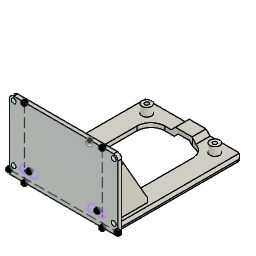
CPU Mount - Blank (Autodesk Fusion 360 design; units mm, degrees)
Autodesk Fusion 360 part; units mm, degrees
note: some values were not read from the file. Set by a fixed rule: which sketch regions a step uses.
sketch "Sketch3" plane through (0, 0, 0) normal (0, 1, 0) x (1, 0, 0)
  line L0 (-39, -50) -> (39, -50)
  line L1 (39, -50) -> (39, 0)
  line L2 (39, 0) -> (-39, 0)
  line L3 (-39, 0) -> (-39, -50)
  line L4 (-56.129, 0) -> (56.129, 0) construction
  circle A0 centre (-36, -47) radius 1.7
  circle A1 centre (-36, -47) radius 3
  circle A2 centre (36, -47) radius 1.7
  circle A3 centre (36, -47) radius 3
  circle A4 centre (-36, -6.7) radius 1.7
  circle A5 centre (-36, -6.7) radius 3
  circle A6 centre (36, -6.7) radius 1.7
  circle A7 centre (36, -6.7) radius 3
  line L5 (-39, -5) -> (39, -5) construction
  dimension "d32" = 50
  dimension "d33" = 78
  dimension "d34" = 39
  dimension "d35" = 3.4
  dimension "d36" = 6
  dimension "d37" = 3.4
  dimension "d38" = 6
  dimension "d39" = 3.4
  dimension "d40" = 6
  dimension "d41" = 3.4
  dimension "d42" = 6
  dimension "d43" = 5
  constraint horizontal L0
  constraint vertical L1
  constraint horizontal L2
  constraint vertical L3
  constraint perpendicular L3 L4
  constraint midpoint origin L4
  constraint collinear L2 L4
  constraint concentric A0 A1
  constraint concentric A2 A3
  constraint concentric A4 A5
  constraint concentric A6 A7
  constraint horizontal A0.centre A2.centre
  constraint vertical A2.centre A6.centre
  constraint vertical A0.centre A4.centre
  constraint horizontal A4.centre A6.centre
  constraint tangent L0 A1
  constraint tangent L3 A1
  constraint tangent L1 A3
  constraint coincident L3 L5.start
  constraint coincident L1 L5.end
  constraint perpendicular L1 L5
  constraint tangent A6 L5
  measures "d32" distance of L0.start L2.end
  measures "d33" distance of L0.start L0.end
  measures "d34" distance of origin L3
  measures "d35" diameter of A0
  measures "d36" diameter of A1
  measures "d37" diameter of A2
  measures "d38" diameter of A3
  measures "d39" diameter of A4
  measures "d40" diameter of A5
  measures "d41" diameter of A6
  measures "d42" diameter of A7
  measures "d43" distance of L1.end L5.end
extrude "Extrude3" add sketch "Sketch3" along normal blind 3 contours A7 | A5 | L0 L1 L2 L3 A1 A3 | A1 | A3
sketch "Sketch4" plane through (0, 3, 0) normal (0, 1, 0) x (-1, 0, 0)
  circle A0 centre (36, 47) radius 1.7
  circle A1 centre (36, 6.7) radius 1.7
  circle A2 centre (-36, 47) radius 1.7
  circle A3 centre (-36, 6.7) radius 1.7
  line L0 (36, 50) -> (-36, 50)
  arc A4 (-36, 50) -> (-39, 47) centre (-36, 47) ccw
  line L1 (-39, 47) -> (-39, 0)
  line L2 (-39, 0) -> (39, 0)
  line L3 (39, 0) -> (39, 47)
  arc A5 (39, 47) -> (36, 50) centre (36, 47) ccw
  line L4 (-39, 3) -> (39, 3) construction
  line L5 (-35.6, 3) -> (35.6, 3)
  line L6 (35.6, 3) -> (35.6, 0)
  line L7 (35.6, 0) -> (-35.6, 0)
  line L8 (-35.6, 0) -> (-35.6, 3)
  line L9 (0, 50) -> (0, 0) construction
  line L10 (35.6, 1.2) -> (33.8, 3)
  line L11 (35.6, 1.2) -> (38.7868, 1.2) construction
  line L12 (-35.6, 1.2) -> (-33.8, 3)
  line L13 (-35.6, 1.2) -> (-32.9375, 1.2) construction
  point P0 (0, 3)
  dimension "d46" = 3
  dimension "d47" = 71.2
  dimension "d48" = 135
  dimension "d49" = 1.2
  dimension "d50" = 45
  dimension "d51" = 1.2
  constraint coincident L1 L4.start
  constraint coincident L3 L4.end
  constraint perpendicular L3 L4
  constraint horizontal L5
  constraint vertical L6
  constraint horizontal L7
  constraint vertical L8
  constraint midpoint L0 L9.start
  constraint coincident L9.end origin
  constraint midpoint L5 P0
  constraint coincident L9 P0
  constraint collinear L2 L7
  constraint collinear L4 L5
  constraint horizontal L11
  constraint coincident L6 L10.start
  constraint coincident L5 L10.end
  constraint horizontal L13
  constraint coincident L8 L12.start
  constraint coincident L4 L12.end
  measures "d46" distance of L2.end L4.end
  measures "d47" distance of L5.start L5.end
  measures "d48" angle of L10 L11
  measures "d49" distance of L6.end L10.start
  measures "d50" angle of L12 L13
  measures "d51" distance of L7.end L12.start
extrude "Extrude4" add sketch "Sketch4" along normal blind 90 contours L2 L5 L6 L7 L8 L10 L12
sketch "Sketch5" plane through (0, 0, 3) normal (0, 0, 1) x (-1, 0, 0)
  line L0 (33.8, -3) -> (-33.8, -3)
  line L1 (-33.8, -3) -> (-33.8, -93)
  line L2 (-33.8, -93) -> (33.8, -93)
  line L3 (33.8, -93) -> (33.8, -3)
  line L4 (0, -3) -> (0, -93) construction
  circle A0 centre (24.5, -26.5) radius 1.45
  circle A1 centre (24.5, -26.5) radius 3.5
  circle A2 centre (24.5, -84.5) radius 1.45
  circle A3 centre (24.5, -84.5) radius 3.5
  circle A4 centre (-24.5, -26.5) radius 1.45
  circle A5 centre (-24.5, -26.5) radius 3.5
  circle A6 centre (-24.5, -84.5) radius 1.45
  circle A7 centre (-24.5, -84.5) radius 3.5
  line L5 (28, -3) -> (-28, -3)
  line L6 (-28, -3) -> (-28, -88) construction
  line L7 (-28, -88) -> (28, -88) construction
  line L8 (28, -88) -> (28, -3) construction
  line L9 (20, -13) -> (-20, -13)
  line L10 (-20, -13) -> (-20, -83)
  line L11 (-20, -83) -> (20, -83)
  line L12 (20, -83) -> (20, -13)
  line L13 (33.8, -48) -> (-33.8, -48) construction
  line L14 (-28.5, -3) -> (-31.5, -3)
  line L15 (-31.5, -3) -> (-31.5, -29)
  line L16 (-31.5, -29) -> (-28.5, -29)
  line L17 (-28.5, -29) -> (-28.5, -3)
  point P0 (0, -88)
  point P1 (-28, -3)
  point P2 (0, -13)
  point P3 (20, -48)
  point P4 (-33.8, -48)
  point P5 (33.8, -48)
  dimension "d54" = 2.9
  dimension "d55" = 7
  dimension "d56" = 2.9
  dimension "d57" = 7
  dimension "d58" = 2.9
  dimension "d59" = 7
  dimension "d60" = 2.9
  dimension "d61" = 7
  dimension "d62" = 58
  dimension "d63" = 49
  dimension "d64" = 23.5
  dimension "d70" = 56
  dimension "d71" = 85
  dimension "d86" = 70
  dimension "d87" = 70
  dimension "d88" = 40
  dimension "d159" = 3
  dimension "d160" = 26
  dimension "d161" = 7
  constraint midpoint L0 L4.start
  constraint midpoint L2 L4.end
  constraint concentric A0 A1
  constraint concentric A2 A3
  constraint concentric A4 A5
  constraint concentric A6 A7
  constraint vertical A0.centre A2.centre
  constraint horizontal A0.centre A4.centre
  constraint horizontal A2.centre A6.centre
  constraint vertical A4.centre A6.centre
  constraint symmetric L4 A2.centre A6.centre
  constraint horizontal L5
  constraint vertical L6
  constraint horizontal L7
  constraint vertical L8
  constraint coincident L0 L5.start
  constraint midpoint L7 P0
  constraint coincident L4 P0
  constraint coincident P1 L5.end
  constraint horizontal L9
  constraint vertical L10
  constraint horizontal L11
  constraint vertical L12
  constraint midpoint L9 P2
  constraint coincident L4 P2
  constraint coincident L12 P3
  constraint midpoint L12 P3
  constraint midpoint L1 P4
  constraint midpoint L3 P5
  constraint coincident P5 L13.start
  constraint coincident P4 L13.end
  constraint coincident P3 L13
  constraint horizontal L14
  constraint vertical L15
  constraint horizontal L16
  constraint vertical L17
  constraint coincident L0 L14.start
  measures "d54" diameter of A0
  measures "d55" diameter of A1
  measures "d56" diameter of A2
  measures "d57" diameter of A3
  measures "d58" diameter of A4
  measures "d59" diameter of A5
  measures "d60" diameter of A6
  measures "d61" diameter of A7
  measures "d62" distance of A0.centre A2.centre
  measures "d63" distance of A2.centre A6.centre
  measures "d64" distance of L0 A0.centre
  measures "d70" distance of L6.end L7.end
  measures "d71" distance of L5.start L7.end
  measures "d86" distance of L9.end L10.end
  measures "d87" distance of L9.start L11.end
  measures "d88" distance of L10.end L11.end
  measures "d159" distance of L14.start L14.end
  measures "d160" distance of L14.start L16.end
  measures "d161" horizontal distance of A4.centre L15.end
extrude "Extrude8" add sketch "Sketch5" along normal blind 38 contours L0 L14 L15 L16 L17
chamfer "Chamfer4" distance 20 distance2 35 1 edges at (30, 29, 41) measured on face at (30.5, 11.6667, 41)
mirror "Mirror1" about plane through (0, 0, 0) normal (1, 0, 0) of "Extrude8"
extrude "Extrude7" cut sketch "Sketch5" against normal blind 3 contours L9 L10 L11 L12
extrude "Extrude5" add sketch "Sketch5" along normal blind 6 contours A1 | A3 | A5 | A7
fillet "Fillet1" radius 3 2 edges at (35.6, 93, 0.6) (-35.6, 93, 0.6)
sketch "Sketch7" plane through (0, 0, 0) normal (0, -1, 0) x (1, 0, 0)
  circle A0 centre (-36, 47) radius 1.7
  circle A1 centre (-36, 6.7) radius 1.7
  circle A2 centre (36, 47) radius 1.7
  circle A3 centre (36, 6.7) radius 1.7
  line L0 (36, 50) -> (-36, 50)
  arc A4 (-36, 50) -> (-39, 47) centre (-36, 47) ccw
  line L1 (-39, 47) -> (-39, 0)
  line L2 (-39, 0) -> (39, 0)
  line L3 (39, 0) -> (39, 47)
  arc A5 (39, 47) -> (36, 50) centre (36, 47) ccw
  line L4 (-28, 50) -> (-28, 0) construction
  line L5 (28, 50) -> (28, 0) construction
  line L6 (19, 50) -> (19, 48.3878)
  line L7 (-39, 3) -> (39, 3) construction
  line L8 (-21, 9) -> (-28, 9)
  line L9 (28, 9) -> (21, 9)
  point P0 (-24.5, 9)
  point P1 (24.5, 9)
  dimension "d72" = 11
  dimension "d73" = 11
  dimension "d74" = 3
  constraint coincident L0 L4.start
  constraint coincident L2 L4.end
  constraint perpendicular L2 L4
  constraint coincident L0 L5.start
  constraint coincident L2 L5.end
  constraint perpendicular L2 L5
  constraint coincident L0 L6.start
  constraint perpendicular L0 L6
  constraint coincident L1 L7.start
  constraint coincident L3 L7.end
  constraint perpendicular L3 L7
  constraint midpoint L8 P0
  constraint midpoint L9 P1
  measures "d72" distance of L1 L4
  measures "d73" distance of L3 L5
  measures "d74" distance of L2 L7
fillet "Fillet2" radius 10 4 edges at (-20, 13, 1.5) (20, 13, 1.5) (-20, 83, 1.5) (20, 83, 1.5)
sketch "Sketch8" plane through (0, 0, 0) normal (0, 0, -1) x (1, 0, 0)
  line L0 (-10, -13) -> (10, -13)
  arc A0 (20, -23) -> (10, -13) centre (10, -23) ccw
  line L1 (20, -23) -> (20, -73)
  arc A1 (10, -83) -> (20, -73) centre (10, -73) ccw
  line L2 (10, -83) -> (-10, -83)
  arc A2 (-20, -73) -> (-10, -83) centre (-10, -73) ccw
  line L3 (-20, -73) -> (-20, -23)
  arc A3 (-10, -13) -> (-20, -23) centre (-10, -23) ccw
  arc A4 (-35.6, -90) -> (-32.6, -93) centre (-32.6, -90) ccw
  line L4 (-32.6, -93) -> (32.6, -93)
  arc A5 (32.6, -93) -> (35.6, -90) centre (32.6, -90) ccw
  line L5 (35.6, -90) -> (35.6, -3)
  line L6 (35.6, -3) -> (39, -3)
  line L7 (39, -3) -> (39, 0)
  line L8 (39, 0) -> (-39, 0)
  line L9 (-39, 0) -> (-39, -3)
  line L10 (-39, -3) -> (-35.6, -3)
  line L11 (-35.6, -3) -> (-35.6, -90)
  line L12 (3.6, -93) -> (3.6, -80.0711) construction
  line L13 (7.6, -93) -> (-0.4, -93)
  line L14 (-0.4, -93) -> (-0.4, -73.9514)
  line L15 (-0.4, -73.9514) -> (7.6, -73.9514)
  line L16 (7.6, -73.9514) -> (7.6, -93)
  dimension "d166" = 8
  dimension "d167" = 32
  constraint coincident L4 L12.start
  constraint perpendicular L4 L12
  constraint horizontal L13
  constraint vertical L14
  constraint horizontal L15
  constraint vertical L16
  constraint coincident L4 L13.start
  measures "d166" distance of L14 L16
  measures "d167" distance of A5.end L12
extrude "Extrude9" cut sketch "Sketch8" against normal blind 2.8 contours L2 L4 L13 L14 L16
sketch "Sketch11" plane through (0, 0, 3) normal (0, 0, 1) x (-1, 0, 0)
  line L0 (28.5, -29) -> (28.5, -3)
  line L1 (28.5, -3) -> (-28.5, -3)
  line L2 (-28.5, -3) -> (-28.5, -29)
  line L3 (-28.5, -29) -> (-31.5, -29)
  line L4 (-31.5, -29) -> (-31.5, -3)
  line L5 (-31.5, -3) -> (-33.8, -3)
  line L6 (-33.8, -3) -> (-33.8, -92.7495)
  arc A0 (-33.8, -92.7495) -> (-32.6, -93) centre (-32.6, -90) ccw
  line L7 (-32.6, -93) -> (32.6, -93)
  arc A1 (32.6, -93) -> (33.8, -92.7495) centre (32.6, -90) ccw
  line L8 (33.8, -92.7495) -> (33.8, -3)
  line L9 (33.8, -3) -> (31.5, -3)
  line L10 (31.5, -3) -> (31.5, -29)
  line L11 (31.5, -29) -> (28.5, -29)
  circle A2 centre (-24.5, -26.5) radius 3.5
  circle A3 centre (24.5, -26.5) radius 3.5
  line L12 (-10, -13) -> (10, -13)
  arc A4 (20, -23) -> (10, -13) centre (10, -23) ccw
  line L13 (20, -23) -> (20, -73)
  arc A5 (10, -83) -> (20, -73) centre (10, -73) ccw
  line L14 (10, -83) -> (-10, -83)
  arc A6 (-20, -73) -> (-10, -83) centre (-10, -73) ccw
  line L15 (-20, -73) -> (-20, -23)
  arc A7 (-10, -13) -> (-20, -23) centre (-10, -23) ccw
  circle A8 centre (24.5, -84.5) radius 3.5
  circle A9 centre (-24.5, -84.5) radius 3.5
  line L16 (-7.6, -83) -> (-7.6, -93)
  line L17 (0.4, -93) -> (0.4, -83)
  line L18 (-9.6, -83) -> (-9.6, -93)
  line L19 (2.4, -93) -> (2.4, -83)
  dimension "d170" = 2
  dimension "d171" = 2
extrude "Extrude10" add sketch "Sketch11" along normal blind 3 contours L7 L14 L17 L19 | L7 L14 L16 L17 | L7 L14 L16 L18
chamfer "Chamfer5" distance 3 angle 45 2 edges at (-2.4, 88, 3) (9.6, 88, 3)
chamfer "Chamfer6" distance 4 angle 45 1 edges at (0, 3, 3)
chamfer "Chamfer7" distance 2.8 angle 45 2 edges at (7.6, 88, 0) (-0.4, 88, 0)
chamfer "Chamfer8" distance 35 distance2 20 1 edges at (-30, 29, 41) measured on face at (-30.5, 29, 15.6667)
sketch "Sketch13" plane through (28.5, 0, 0) normal (-1, 0, 0) x (0, -1, 0)
  line L0 (-7, 3) -> (-3, 7)
  line L1 (-3, 7) -> (-3, 41)
  line L2 (-3, 41) -> (-9, 41)
  line L3 (-9, 41) -> (-29, 6)
  line L4 (-29, 6) -> (-29, 3)
  line L5 (-29, 3) -> (-7, 3)
  line L6 (-3, 41) -> (-10.7143, 41)
  line L7 (-10.7143, 41) -> (-10.7143, 38)
  line L8 (-10.7143, 38) -> (-3, 38)
  line L9 (-3, 38) -> (-3, 41)
  dimension "d311" = 3
  constraint horizontal L6
  constraint vertical L7
  constraint horizontal L8
  constraint vertical L9
  constraint coincident L1.end L2.start
  constraint coincident L3 L7.end
  measures "d311" distance of L1.end L8.end
extrude "Extrude12" add sketch "Sketch13" along normal up to surface (57 mm away) contours L1 L2 L3 L6 L8 L9
sketch "Sketch14" plane through (0, 3, 0) normal (0, 1, 0) x (-1, 0, 0)
  line L0 (28.5, 38) -> (-28.5, 38)
  line L1 (-28.5, 38) -> (-28.5, 7)
  line L2 (-28.5, 7) -> (28.5, 7)
  line L3 (28.5, 7) -> (28.5, 38)
  line L4 (-10.85, 38) -> (-9.15, 38)
  line L5 (-9.15, 38) -> (-9.15, 12.3)
  line L6 (-9.15, 12.3) -> (-10.85, 12.3)
  line L7 (-10.85, 12.3) -> (-10.85, 38)
  line L8 (7.15, 38) -> (9.05, 38)
  line L9 (9.05, 38) -> (9.05, 12.3)
  line L10 (9.05, 12.3) -> (7.15, 12.3)
  line L11 (7.15, 12.3) -> (7.15, 38)
  constraint horizontal L4
  constraint vertical L5
  constraint horizontal L6
  constraint vertical L7
  constraint coincident L0 L4.start
  constraint horizontal L8
  constraint vertical L9
  constraint horizontal L10
  constraint vertical L11
  constraint coincident L0 L8.start
  constraint collinear L6 L10
extrude "Extrude13" add sketch "Sketch14" along normal blind 7.8 contours L0 L8 L9 L10 L11 | L0 L4 L5 L6 L7
fillet "Fillet4" radius 5 2 edges at (-31.5, 6, 41) (31.5, 6, 41)
fillet "Fillet5" radius 3 2 edges at (28.5, 6.8571, 38) (-28.5, 6.8571, 38)
extrude "Extrude14" cut 1 faces at (-11.4895, 0, 33.3208) along direction (0, 1, 0) blind 0.2
equation "d34 = d33 / 2"
equation "d37 = d35"
equation "d38 = d36"
equation "d39 = d35"
equation "d40 = d36"
equation "d41 = d35"
equation "d42 = d36"
equation "d56 = d54"
equation "d57 = d55"
equation "d58 = d54"
equation "d59 = d55"
equation "d60 = d54"
equation "d61 = d55"
